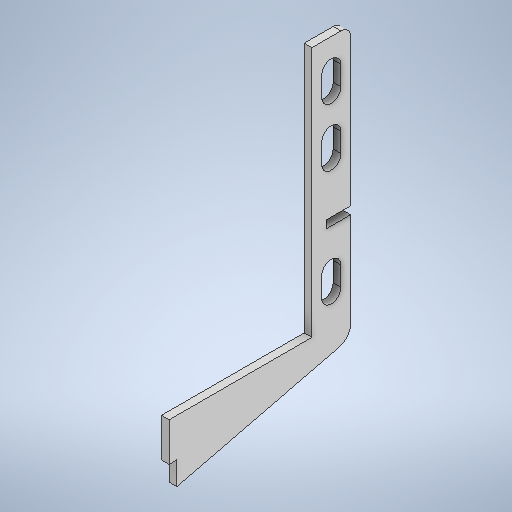
# Autodesk Inventor part: battery front brace
Saved by Autodesk Inventor 2025.2 (Build 292293000, 293)
## iProperties
Created: 2025-01-25
Part Number: battery front brace
Material: Generic
Document SubType Name: Modeling
Designer: alex
Density: 1 g/cm^3
Appearance: Default
Author: alex
Autodesk Inventor part; units mm, degrees
ref_plane "YZ Plane" through (0, 0, 0) normal (1, 0, 0) x (0, 1, 0)
ref_plane "XZ Plane" through (0, 0, 0) normal (0, 1, 0) x (-1, 0, 0)
ref_plane "XY Plane" through (0, 0, 0) normal (0, 0, 1) x (1, 0, 0)
sketch "Sketch1" plane through (0, 0, 0) normal (1, 0, 0) x (0, 1, 0)
  line L0 (0, 0) -> (50.8, 0)
  line L1 (50.8, 0) -> (50.8, -187.96)
  line L2 (50.8, -187.96) -> (381, -187.96)
  line L3 (381, -187.96) -> (381, -226.06)
  line L4 (0, 0) -> (0, -10.16)
  line L5 (0, -10.16) -> (-30.48, -10.16)
  line L6 (-30.48, -10.16) -> (21.8491, -224.2335)
  line L7 (40.3542, -238.76) -> (368.3, -238.76)
  line L8 (342.9, -200.66) -> (317.5, -200.66)
  line L9 (304.8, -213.36) -> (304.8, -213.36)
  line L10 (317.5, -226.06) -> (342.9, -226.06)
  line L11 (355.6, -213.36) -> (355.6, -213.36)
  line L12 (266.7, -200.66) -> (241.3, -200.66)
  line L13 (228.6, -213.36) -> (228.6, -213.36)
  line L14 (241.3, -226.06) -> (266.7, -226.06)
  line L15 (279.4, -213.36) -> (279.4, -213.36)
  line L16 (152.4, -213.36) -> (152.4, -213.36)
  line L17 (203.2, -213.36) -> (203.2, -213.36)
  line L18 (114.3, -200.66) -> (88.9, -200.66)
  line L19 (76.2, -213.36) -> (76.2, -213.36)
  line L20 (88.9, -226.06) -> (114.3, -226.06)
  line L21 (127, -213.36) -> (127, -213.36)
  line L22 (127, -226.06) -> (152.4, -226.06)
  line L23 (203.2, -226.06) -> (228.6, -226.06)
  line L24 (279.4, -226.06) -> (304.8, -226.06)
  line L25 (355.6, -226.06) -> (381, -226.06)
  line L26 (355.6, -226.06) -> (355.6, -238.76)
  arc A0 (355.6, -213.36) -> (342.9, -200.66) centre (342.9, -213.36) ccw
  arc A1 (342.9, -226.06) -> (355.6, -213.36) centre (342.9, -213.36) ccw
  arc A2 (317.5, -200.66) -> (304.8, -213.36) centre (317.5, -213.36) ccw
  arc A3 (304.8, -213.36) -> (317.5, -226.06) centre (317.5, -213.36) ccw
  arc A4 (279.4, -213.36) -> (266.7, -200.66) centre (266.7, -213.36) ccw
  arc A5 (266.7, -226.06) -> (279.4, -213.36) centre (266.7, -213.36) ccw
  arc A6 (241.3, -200.66) -> (228.6, -213.36) centre (241.3, -213.36) ccw
  arc A7 (228.6, -213.36) -> (241.3, -226.06) centre (241.3, -213.36) ccw
  arc A8 (127, -213.36) -> (114.3, -200.66) centre (114.3, -213.36) ccw
  arc A9 (88.9, -200.66) -> (76.2, -213.36) centre (88.9, -213.36) ccw
  arc A10 (76.2, -213.36) -> (88.9, -226.06) centre (88.9, -213.36) ccw
  arc A11 (114.3, -226.06) -> (127, -213.36) centre (114.3, -213.36) ccw
  arc A12 (21.8491, -224.2335) -> (40.3542, -238.76) centre (40.3542, -219.71) ccw
  arc A13 (368.3, -238.76) -> (381, -226.06) centre (368.3, -226.06) ccw
  line L27 (165.1, -238.76) -> (165.1, -207.01)
  line L28 (165.1, -207.01) -> (175.26, -207.01)
  line L29 (175.26, -207.01) -> (175.26, -238.76)
  point P0 (381, -238.76)
  point P1 (355.6, -200.66)
  point P2 (279.4, -200.66)
  point P3 (203.2, -200.66)
  point P4 (127, -200.66)
  point P5 (76.2, -226.06)
  point P6 (127, -213.36)
  point P7 (76.2, -213.36)
  point P8 (228.6, -213.36)
  point P9 (355.6, -213.36)
  point P10 (304.8, -213.36)
  dimension "d0" = 50.8
  dimension "d1" = 187.96
  dimension "d2" = 330.2
  dimension "d3" = 50.8
  dimension "d5" = 10.16
  dimension "d6" = 30.48
  dimension "d10" = 50.8
  dimension "d11" = 25.4
  dimension "d12" = 25.4
  dimension "d13" = 12.7
  dimension "d14" = 12.7
  dimension "d15" = 50.8
  dimension "d16" = 50.8
  dimension "d17" = 50.8
  dimension "d18" = 12.7
  dimension "d19" = 19.05
  dimension "d22" = 12.7
  dimension "d24" = 12.7
  dimension "d25" = 10.16
  dimension "d26" = 31.75
  dimension "d27" = 114.3
  dimension "d28" = 196.85
  constraints: 60 end point, 32 point on line, 28 point on circle, 28 tangent, 14 centre point, 12 perpendicular, 10 equal radius, 9 equal length, 5 horizontal, 3 collinear, 1 vertical
  measures "d0" distance of L0.start L0.end
  measures "d1" distance of L0.end L1.end
  measures "d2" distance of L1.end L2.end
  measures "d3" distance of L2.end point (381, -238.76)
  measures "d5" distance of L0.start L4.end
  measures "d6" distance of L4.end L5.end
  measures "d10" distance of L24.end L25.start
  measures "d11" distance of L25.start L25.end
  measures "d12" distance of L25.start point (355.6, -200.66)
  measures "d13" distance of L25.start L26.end
  measures "d14" radius of A0
  measures "d15" distance of L23.end L24.start
  measures "d16" distance of L22.end L23.start
  measures "d17" distance of point (76.2, -226.06) L22.start
  measures "d18" radius of A4
  measures "d19" radius of A12
  measures "d22" radius of A13
  measures "d24" distance between parallel lines of L2 L18
  measures "d25" distance of L27.end L28.end
  measures "d26" distance of L28.end L29.end
  measures "d27" distance between parallel lines of L1 L27
  measures "d28" distance between parallel lines of L5 L28
extrude "Extrusion1" add sketch "Sketch1" along normal blind 10.16 contours L0 L1 L2 L3 L25 L26 L7 L29 L28 L27 A12 L6 L5 L4 | A13 L7 L26 L25
body "Solid1"
